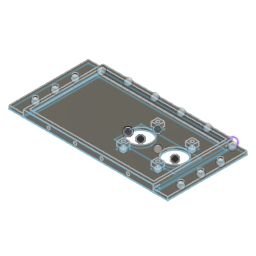
Side-Panel-120x60mm (Autodesk Fusion 360 design; units mm, degrees)
part number: 2026-04-12-13-41-56-896
Autodesk Fusion 360 part; units mm, degrees
sketch "Sketch1" plane through (0, 0, 0) normal (0, 0, 1) x (1, 0, 0)
  line L0 (60, 30) -> (-60, 30)
  line L1 (-60, 30) -> (-60, -30)
  line L2 (-60, -30) -> (60, -30)
  line L3 (60, -30) -> (60, 30)
  line L4 (-50, 30) -> (-50, -30)
  line L5 (50, 30) -> (50, -30)
  circle A0 centre (-55, 15) radius 1.75
  circle A1 centre (-55, 0) radius 1.75
  circle A2 centre (-55, -15) radius 1.75
  circle A3 centre (55, 15) radius 1.75
  circle A4 centre (55, 0) radius 1.75
  circle A5 centre (55, -15) radius 1.75
  line L6 (-49, 25) -> (49, 25)
  line L7 (-49, -25) -> (49, -25)
  line L8 (-49, 30) -> (-49, 25)
  line L9 (-49, -25) -> (-49, -30)
  line L10 (49, 30) -> (49, 25)
  line L11 (49, -25) -> (49, -30)
  line L12 (-49, -25) -> (-49, 25)
  line L13 (-47, -25) -> (-47, 25)
  line L14 (49, -25) -> (49, 25)
  line L15 (47, -25) -> (47, 25)
  line L16 (45, 10) -> (0, 10)
  line L17 (0, 10) -> (0, -10)
  line L18 (0, -10) -> (45, -10)
  line L19 (45, -10) -> (45, 10)
  circle A6 centre (9.5, 0) radius 8.25
  circle A7 centre (35.5, 0) radius 8.25
  circle A8 centre (9.5, 13) radius 1.15
  line L20 (12, 10.5) -> (7, 10.5)
  line L21 (7, 10.5) -> (7, 15.5)
  line L22 (7, 15.5) -> (12, 15.5)
  line L23 (12, 15.5) -> (12, 10.5)
  line L24 (33, 15.5) -> (38, 15.5)
  line L25 (38, 10.5) -> (33, 10.5)
  line L26 (33, 10.5) -> (33, 15.5)
  circle A9 centre (35.5, 13) radius 1.15
  line L27 (38, 15.5) -> (38, 10.5)
  line L28 (12, -10.5) -> (12, -15.5)
  circle A10 centre (9.5, -13) radius 1.15
  line L29 (33, -15.5) -> (33, -10.5)
  circle A11 centre (35.5, -13) radius 1.15
  line L30 (33, -10.5) -> (38, -10.5)
  line L31 (38, -10.5) -> (38, -15.5)
  line L32 (38, -15.5) -> (33, -15.5)
  line L33 (7, -10.5) -> (12, -10.5)
  line L34 (7, -15.5) -> (7, -10.5)
  line L35 (12, -15.5) -> (7, -15.5)
  point P0 (22.5, 0)
  point P1 (9.5, 0)
  point P2 (35.5, 0)
  point P3 (9.5, 13)
  dimension "d25" = 16.5
  dimension "d26" = 16.5
  constraint horizontal L0
  constraint perpendicular L0 L1
  constraint parallel L0 L2
  constraint parallel L1 L3
  constraint coincident L2 L4.end
  constraint perpendicular L2 L4
  constraint coincident L0 L5.start
  constraint coincident L2 L5.end
  constraint perpendicular L2 L5
  constraint coincident L0 L8.start
  constraint coincident L2 L9.end
  constraint perpendicular L2 L9
  constraint coincident L2 L11.end
  constraint perpendicular L2 L11
  constraint perpendicular L6 L10
  constraint perpendicular L7 L11
  constraint collinear L8 L9
  constraint collinear L10 L11
  constraint coincident L7 L13.start
  constraint coincident L6 L13.end
  constraint perpendicular L6 L13
  constraint coincident L7 L15.start
  constraint coincident L6 L15.end
  constraint perpendicular L6 L15
  constraint horizontal L16
  constraint perpendicular L16 L17
  constraint parallel L16 L18
  constraint parallel L17 L19
  constraint coincident P1 A6.centre
  constraint coincident P2 A7.centre
  constraint horizontal L20
  constraint perpendicular L20 L21
  constraint parallel L20 L22
  constraint parallel L21 L23
  constraint coincident P3 A8.centre
  constraint horizontal L25
  constraint perpendicular L25 L26
  constraint parallel L24 L25
  constraint parallel L26 L27
  constraint horizontal L35
  constraint perpendicular L34 L35
  constraint parallel L33 L35
  constraint parallel L28 L34
  constraint horizontal L32
  constraint perpendicular L29 L32
  constraint parallel L30 L32
  constraint parallel L29 L31
  measures "d25" diameter of A6
  measures "d26" diameter of A7
extrude "Extrude9" add sketch "Sketch1" along normal blind 5 contours L20 L21 L22 L23 | L24 L25 L26 L27 | L28 L33 L34 L35 | L29 L30 L31 L32 makes body 1 at (36.0246, 14.0234, 3.3333) makes body 2 at (10.6486, -13.0573, 3.3333) makes body 3 at (10.6486, 12.9427, 3.3333) makes body 4 at (36.0246, -11.9766, 3.3333)
extrude "Extrude10" add sketch "Sketch1" along normal blind 2 separate body contours L6 L7 L13 L15 | L16 L17 L18 L19 makes body 5
extrude "Extrude1" add sketch "Sketch1" along normal blind 2.5 separate body contours L0 L2 L3 L5 | L0 L2 L5 L10 L11 L14 | L0 L2 L4 L8 L9 L12 | L6 L7 L14 L15 | L0 L1 L2 L4 | L6 L7 L12 L13 makes body 6 at (54.7103, -23.915, 0) makes body 7 at (-54.7103, -23.915, 0)
sketch "Sketch2" plane through (0, 0, 2.5) normal (0, 0, 1) x (-1, 0, 0)
  circle A0 centre (-55, 0) radius 1.75
  circle A1 centre (55, -15) radius 1.75
  circle A2 centre (55, 15) radius 1.75
  circle A3 centre (55, 0) radius 1.75
  circle A4 centre (-55, 15) radius 1.75
  circle A5 centre (-55, -15) radius 1.75
  line L0 (-60, 30) -> (-60, -30)
  line L1 (-60, -30) -> (-49, -30)
  line L2 (60, -30) -> (60, 30)
  line L3 (-49, 30) -> (-60, 30)
  line L4 (-47, 25) -> (-49, 25)
  line L5 (-49, 25) -> (-49, 30)
  line L6 (-49, -30) -> (-49, -25)
  line L7 (-49, -25) -> (-47, -25)
  line L8 (49, -25) -> (49, -30)
  line L9 (49, -30) -> (60, -30)
  line L10 (60, 30) -> (49, 30)
  line L11 (49, 30) -> (49, 25)
  line L12 (-47, -25) -> (-47, 25)
  line L13 (49, 25) -> (47, 25)
  line L14 (47, 25) -> (47, -25)
  line L15 (47, -25) -> (49, -25)
extrude "Extrude2" add sketch "Sketch1" along normal blind 5 separate body contours L0 L6 L8 L10 | L6 L7 L14 L15 | L2 L7 L9 L11 | L6 L7 L12 L13 makes body 8
sketch "Sketch3" plane through (0, -30, 0) normal (0, -1, 0) x (1, 0, 0)
  line L0 (-49, 0) -> (49, 0)
  line L1 (49, 0) -> (49, 5)
  line L2 (49, 5) -> (-49, 5)
  line L3 (-49, 5) -> (-49, 0)
  circle A0 centre (30, 2.5) radius 1.2
  circle A1 centre (10, 2.5) radius 1.15
  circle A2 centre (-10, 2.5) radius 1.2
  circle A3 centre (-30, 2.5) radius 1.15
extrude "Extrude3" cut sketch "Sketch3" against normal blind 3 contours A0 | A1 | A2 | A3 bodies 8
sketch "Sketch4" plane through (0, 30, 0) normal (0, 1, 0) x (-1, 0, 0)
  line L0 (-49, 0) -> (49, 0)
  line L1 (49, 0) -> (49, 5)
  line L2 (49, 5) -> (-49, 5)
  line L3 (-49, 5) -> (-49, 0)
  circle A0 centre (-30, 2.5) radius 1.15
  circle A1 centre (-10, 2.5) radius 1.15
  circle A2 centre (30, 2.5) radius 1.2
  circle A3 centre (10, 2.5) radius 1.2
  point P0 (-49, 2.5)
  dimension "d38" = 2.3
  measures "d38" diameter of A0
extrude "Extrude4" cut sketch "Sketch4" against normal blind 3 contours A0 | A1 | A2 | A3 bodies 8
chamfer "Chamfer1" distance 2.5 angle 45 2 edges at (0, 25, 5) (0, -25, 5) on bodies 8
extrude "Extrude11" add sketch "Sketch1" along normal blind 1.5 contours A8 | A9 | A10 | A11 bodies 1 2 3 4 5 6 7 8
